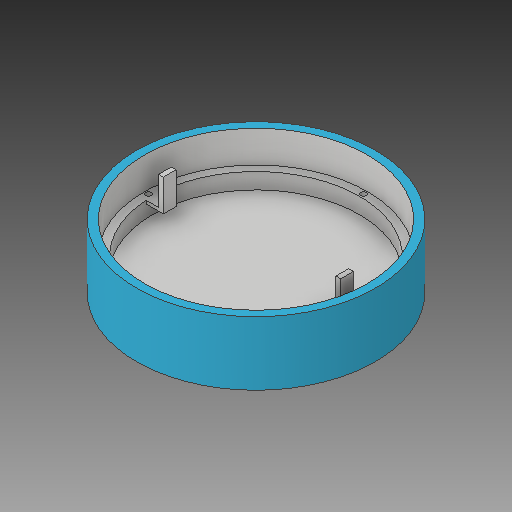
# Autodesk Inventor part: 바텀(하)
Saved by Autodesk Inventor 2019 (Build 230136000, 136)
## iProperties
Created: 2018-04-02
Part Number: 바텀(하)
Material: 일반
Document SubType Name: Modeling
Designer: CK
Density: 1 g/cm^3
Appearance: 기본값
Mass: 265.772 g
Surface Area: 694.673 cm^2
Volume: 265.772 cm^3
Author: CK
Autodesk Inventor part; units mm, degrees
ref_plane "XZ Plane" through (0, 0, 0) normal (0, 1, 0) x (-1, 0, 0)
ref_plane "XY Plane" through (0, 0, 0) normal (0, 0, 1) x (1, 0, 0)
sketch "스케치1" plane through (0, 0, 0) normal (0, 1, 0) x (-1, 0, 0)
  circle A0 centre (0, 0) radius 75
  dimension "d0" = 150
  constraints: 1 centre point, 1 coincident
  measures "d0" diameter of A0
extrude "돌출1" add sketch "스케치1" along normal blind 40
shell "쉘1" thickness 10 removed faces 1 at (17.2828, 40, 11.7077)
sketch "스케치6" plane through (0, 40, 0) normal (0, 1, 0) x (1, 0, 0)
  circle A0 centre (0, 0) radius 65
  circle A1 centre (0, 0) radius 70
  dimension "d22" = 130
  dimension "d23" = 140
  constraints: 2 centre point, 2 coincident
  measures "d22" diameter of A0
  measures "d23" diameter of A1
extrude "돌출5" cut sketch "스케치6" against normal blind 20
sketch "스케치8" plane through (0, 0, 0) normal (0, -1, 0) x (1, 0, 0)
  circle A0 centre (0, 0) radius 67.5
  point P0 (0, -67.5)
  point P1 (67.5, 0)
  point P2 (0, 67.5)
  point P3 (-67.5, 0)
  dimension "d31" = 135
  constraints: 4 point on circle, 1 centre point, 1 coincident
  measures "d31" diameter of A0
hole "구멍2" at (0, 0, -67.5) at (67.5, 0, 0) at (0, 0, 67.5) at (-67.5, 0, 0) direction (0, 1, 0) diameter 3.5 depth 25 counterbore diameter 6.7 counterbore depth 9
ref_plane "작업 평면1" through (57, 0, 0) normal (1, 0, 0) x (0, 1, 0)
sketch "스케치10" plane through (57, 0, 0) normal (1, 0, 0) x (0, 1, 0)
  line L0 (38, -4.2173) -> (18, -4.2173)
  line L1 (18, -4.2173) -> (18, 3.7827)
  line L2 (18, 3.7827) -> (38, 3.7827)
  line L3 (38, 3.7827) -> (38, -4.2173)
  line L4 (38, -4.2173) -> (18, 3.7827) construction
  line L5 (18, -4.2173) -> (38, 3.7827) construction
  line L6 (10, 65) -> (10, -65) projected
  point P0 (0, 0)
  point P1 (28, -0.2173)
  dimension "d40" = 20
  dimension "d41" = 8
  dimension "d42" = 18
  constraints: 12 end point, 2 midpoint, 2 parallel, 1 horizontal, 1 perpendicular
  measures "d40" distance of L1.end L2.end
  measures "d41" distance of L2.end L0.start
  measures "d42" distance from line of L6 point (28, -0.217)
extrude "돌출6" add sketch "스케치10" against normal blind 3
sketch "스케치11" plane through (57, 0, 0) normal (1, 0, 0) x (0, 0, -1)
  line L0 (4.2173, 38) -> (4.2173, 18) projected
  line L1 (4.2173, 18) -> (-3.7827, 18)
  line L2 (-3.7827, 18) -> (-3.7827, 20)
  line L3 (-3.7827, 20) -> (4.2173, 20)
  line L4 (4.2173, 20) -> (4.2173, 18)
  point P0 (0, 0)
  dimension "d45" = 8
  dimension "d46" = 2
  constraints: 8 end point, 2 parallel, 1 horizontal, 1 perpendicular
  measures "d45" distance of L2.end L3.end
  measures "d46" distance of L1.end L2.end
extrude "돌출7" add sketch "스케치11" along normal up to next
pattern_circular "원형 패턴1" count 2 over 360 about axis through (0, 0, 0) along (0, 1, 0) of "돌출6", "돌출7"
